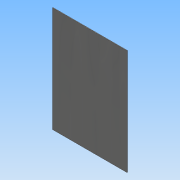
# Autodesk Inventor part: LCD12864-large-film
Saved by Autodesk Inventor 2016 (Build 200138000, 138)
## iProperties
Created: 2015-10-22
Part Number: LCD12864-large-film
Material: Generic
Document SubType Name: Modeling
Designer: Openlab
Density: 1 g/cm^3
Appearance: Light Gray
Author: Openlab
Autodesk Inventor part; units mm, degrees
ref_plane "YZ Plane" through (0, 0, 0) normal (1, 0, 0) x (0, 1, 0)
ref_plane "XZ Plane" through (0, 0, 0) normal (0, 1, 0) x (-1, 0, 0)
ref_plane "XY Plane" through (0, 0, 0) normal (0, 0, 1) x (1, 0, 0)
sketch "Sketch1" plane through (0, 0, 0) normal (0, 1, 0) x (-1, 0, 0)
  line L0 (24.25, 34.35) -> (-24.25, 34.35)
  line L1 (-24.25, 34.35) -> (-24.25, -34.35)
  line L2 (-24.25, -34.35) -> (24.25, -34.35)
  line L3 (24.25, -34.35) -> (24.25, 34.35)
  line L4 (-24.25, 34.35) -> (24.25, -34.35) construction
  line L5 (-24.25, -34.35) -> (24.25, 34.35) construction
  point P0 (0, 0)
  point P1 (0, 0)
  dimension "d0" = 68.7
  dimension "d1" = 48.5
  constraints: 12 end point, 2 parallel, 1 coincident, 1 horizontal, 1 midpoint, 1 perpendicular
  measures "d0" distance of L2.end L0.start
  measures "d1" distance of L1.end L2.end
extrude "Extrusion1" add sketch "Sketch1" along normal blind 0.3
body "Solid1"
